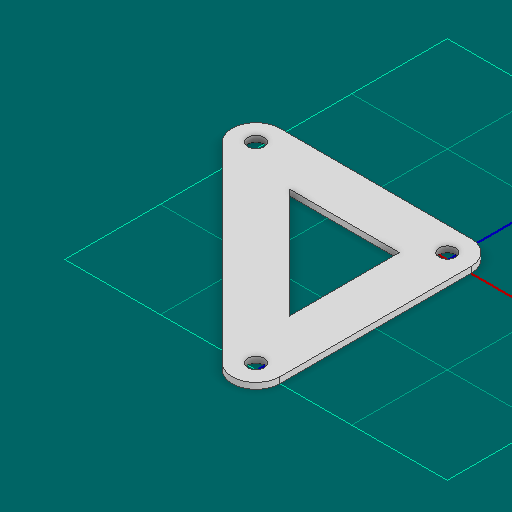
# Autodesk Inventor part: triangle_gusset
Saved by Autodesk Inventor 2025 (Build 290162000, 162)
## iProperties
Created: 2024-10-07
Part Number: triangle_gusset
Material: Generic
Document SubType Name: Modeling
Designer: averey
Density: 1 g/cm^3
Appearance: Default
Author: averey
Autodesk Inventor part; units mm, degrees
ref_plane "YZ Plane" through (0, 0, 0) normal (1, 0, 0) x (0, 1, 0)
ref_plane "XZ Plane" through (0, 0, 0) normal (0, 1, 0) x (-1, 0, 0)
ref_plane "XY Plane" through (0, 0, 0) normal (0, 0, 1) x (1, 0, 0)
sketch "main" plane through (0, 0, 0) normal (0, 0, 1) x (1, 0, 0)
  circle A0 centre (-25.7384, -24.2854) radius 2.1844
  circle A1 centre (-25.7384, 26.5146) radius 2.1844
  circle A2 centre (25.0616, -24.2854) radius 2.1844
  arc A3 (-32.0884, -24.2854) -> (-25.7384, -30.6354) centre (-25.7384, -24.2854) ccw
  arc A4 (25.0616, -30.6354) -> (29.5518, -19.7953) centre (25.0616, -24.2854) ccw
  arc A5 (-21.2482, 31.0047) -> (-32.0884, 26.5146) centre (-25.7384, 26.5146) ccw
  line L0 (-25.7384, -30.6354) -> (25.0616, -30.6354)
  line L1 (-32.0884, -24.2854) -> (-32.0884, 26.5146)
  line L2 (29.5518, -19.7953) -> (-21.2482, 31.0047)
  line L3 (-19.3884, 11.1843) -> (9.7314, -17.9354)
  line L4 (9.7314, -17.9354) -> (-19.3884, -17.9354)
  line L5 (-19.3884, -17.9354) -> (-19.3884, 11.1843)
  point P0 (-9.8909, -6.4767)
  point P1 (-28.0498, 28.318)
  dimension "d0" = 12.7
  dimension "d1" = 12.7
  dimension "d2" = 12.7
  dimension "d5" = 12.7
  measures "d0" diameter of A3
  measures "d1" diameter of A4
  measures "d2" diameter of A5
  measures "d5" distance between parallel lines of L2 L3
sketch "Sketch1" plane through (0, 0, 0) normal (0, 1, 0) x (-1, 0, 0)
  circle A0 centre (0, 0) radius 2.1844
  circle A1 centre (0, 50.8) radius 2.1844
  circle A2 centre (50.8, 0) radius 2.1844
  arc A3 (-6.35, 0) -> (0, -6.35) centre (0, 0) ccw
  arc A4 (50.8, -6.35) -> (55.2901, 4.4901) centre (50.8, 0) ccw
  arc A5 (4.4901, 55.2901) -> (-6.35, 50.8) centre (0, 50.8) ccw
  line L0 (0, -6.35) -> (50.8, -6.35)
  line L1 (-6.35, 0) -> (-6.35, 50.8)
  line L2 (55.2901, 4.4901) -> (4.4901, 55.2901)
  line L3 (6.35, 35.4697) -> (35.4697, 6.35)
  line L4 (35.4697, 6.35) -> (6.35, 6.35)
  line L5 (6.35, 6.35) -> (6.35, 35.4697)
  constraints: 1 other
extrude "Extrusion1" add sketch "Sketch1" along normal blind 1.5875
body "Solid1"
